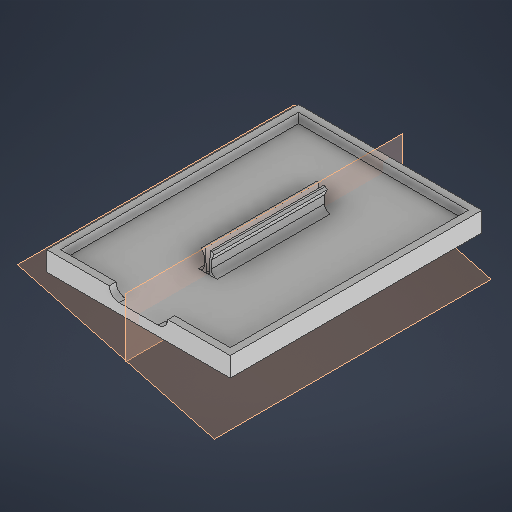
# Autodesk Inventor part: Bolt Slot Covers
Saved by Autodesk Inventor 2026.2 (Build 302298000, 298)
## iProperties
Created: 2026-05-27
Part Number: Bolt Slot Covers
Material: Generic
Document SubType Name: Modeling
Designer: mayhe
Density: 1 g/cm^3
Appearance: Default
Author: mayhe
Autodesk Inventor part; units mm, degrees
ref_plane "XZ Plane" through (0, 0, 0) normal (0, 1, 0) x (-1, 0, 0)
ref_plane "XY Plane" through (0, 0, 0) normal (0, 0, 1) x (1, 0, 0)
sketch "Sketch1" plane through (0, 0, 0) normal (0, 1, 0) x (-1, 0, 0)
  line L0 (47, 64.5) -> (-47, 64.5)
  line L1 (-47, 64.5) -> (-47, -64.5)
  line L2 (-47, -64.5) -> (47, -64.5)
  line L3 (47, -64.5) -> (47, 64.5)
  line L4 (47, 64.5) -> (-47, -64.5) construction
  line L5 (-47, 64.5) -> (47, -64.5) construction
  point P0 (0, 0)
  dimension "d0" = 94
  dimension "d1" = 129
  constraints: 12 end point, 2 midpoint, 2 parallel, 1 horizontal, 1 perpendicular
  measures "d0" distance of L2.end L1.end
  measures "d1" distance of L1.end L0.end
extrude "Base" add sketch "Sketch1" along normal mid plane 5
sketch "Sketch6" plane through (0, 2.5, 0) normal (0, 1, 0) x (1, 0, 0)
  line L0 (-47, -64.5) -> (47, -64.5) projected
  line L1 (-47, 64.5) -> (-47, -64.5) projected
  line L2 (-47, -64.5) -> (47, -64.5) projected
  line L3 (47, -64.5) -> (47, 64.5) projected
  line L4 (47, 64.5) -> (-47, 64.5) projected
  line L5 (-43.5, -61) -> (-43.5, 61)
  line L6 (-43.5, 61) -> (43.5, 61)
  line L7 (43.5, 61) -> (43.5, -61)
  line L8 (43.5, -61) -> (-43.5, -61)
  line L9 (0, -61) -> (0, -64.5)
  line L10 (-15, -61) -> (15, -61)
  line L11 (15, -61) -> (15, -64.5)
  line L12 (15, -64.5) -> (-15, -64.5)
  line L13 (-15, -64.5) -> (-15, -61)
  line L14 (-15, -61) -> (15, -64.5) construction
  line L15 (15, -61) -> (-15, -64.5) construction
  point P0 (0, 0)
  point P1 (0, -62.75)
  point P2 (-15, -61)
  point P3 (15, -61)
  point P4 (15, -64.5)
  point P5 (47, -64.5)
  dimension "d31" = 3.5
  dimension "d32" = 30
  constraints: 22 end point, 5 midpoint, 2 parallel, 1 horizontal, 1 perpendicular, 1 point on line, 3 other
  measures "d31" distance between parallel lines of L1 L5
  measures "d32" distance of L11.end L12.end
extrude "Walls" add sketch "Sketch6" along normal blind 5 contours L1 L4 L3 L0 L11 L8 L7 L6 L5 L13
sketch "Sketch7" plane through (0, 2.5, 0) normal (0, 1, 0) x (1, 0, 0)
  line L0 (0, 29) -> (0, -29) construction
  line L1 (-1.75, 29) -> (-1.75, -29)
  line L2 (1.75, -29) -> (1.75, 29)
  arc A0 (1.75, 29) -> (-1.75, 29) centre (0, 29) ccw
  arc A1 (-1.75, -29) -> (1.75, -29) centre (0, -29) ccw
  line L3 (1.75, -29) -> (-1.75, -29)
  line L4 (-1.75, 29) -> (1.75, 29)
  point P0 (0, 0)
  dimension "d35" = 29
  dimension "d36" = 3.5
  constraints: 12 end point, 4 point on circle, 4 tangent, 2 centre point, 2 parallel, 1 horizontal, 1 midpoint, 1 vertical
  measures "d35" distance of point (0, 0) L0.end
  measures "d36" diameter of A1
extrude "Extrusion7" add sketch "Sketch7" along normal blind 7 contours L4 L2 L3 L1
sketch "Sketch8" plane through (0, 9.5, 0) normal (0, 1, 0) x (1, 0, 0)
  line L0 (1.75, -29) -> (1.75, 29) projected
  line L1 (-1.75, 29) -> (-1.75, -29) projected
  arc A0 (-3.25, -29) -> (3.25, -29) centre (0, -29) ccw
  line L2 (-3.25, -29) -> (-3.25, 29)
  arc A1 (3.25, 29) -> (-3.25, 29) centre (0, 29) ccw
  line L3 (3.25, 29) -> (3.25, -29)
  line L4 (1.75, 29) -> (-1.75, 29) projected
  line L5 (-1.75, -29) -> (1.75, -29) projected
  line L6 (-3.25, -29) -> (3.25, -29)
  line L7 (-3.25, 29) -> (3.25, 29)
  point P0 (0, 0)
  constraints: 8 end point, 4 point on circle, 2 centre point, 1 horizontal, 1 parallel
extrude "Knob Width" add sketch "Sketch8" along normal blind 4 contours L5 L1 L4 L0 | L0 L7 L3 L6 | L6 L2 L7 L1
chamfer "Chamfer3" distance 1.5 distance2 3 2 edges at (-3.25, 9.5, 0) (3.25, 9.5, 0) measured on face at (2.75, 9.5, 0) measured on face at (-2.75, 9.5, 0)
chamfer "Chamfer4" distance 1 distance2 1 2 edges at (-3.25, 13.5, 0) (3.25, 13.5, 0) measured on face at (-2.75, 13.5, 0) measured on face at (2.75, 13.5, 0)
fillet "Fillet3" radius 3 2 edges at (1.75, 2.5, 0) (-1.75, 2.5, 0)
sketch "Sketch9" plane through (0, 13.5, 0) normal (0, 1, 0) x (1, 0, 0)
  line L0 (-0.625, 37.5) -> (0.625, 37.5)
  line L1 (0.625, 37.5) -> (0.625, -37.5)
  line L2 (0.625, -37.5) -> (-0.625, -37.5)
  line L3 (-0.625, 37.5) -> (0.625, -37.5) construction
  line L4 (0.625, 37.5) -> (-0.625, -37.5) construction
  line L5 (0, -32.25) -> (0, 0)
  line L6 (-1.75, 29) -> (-1.75, -29) projected
  line L7 (-0.625, -37.5) -> (-0.625, 37.5)
  point P0 (0.125, -28.4242)
  constraints: 14 end point, 3 parallel, 2 midpoint, 1 horizontal, 1 perpendicular
extrude "Extrusion9" cut sketch "Sketch9" against normal up to surface (11 mm away)
fillet "Fillet5" radius 5 2 edges at (-15, 2.5, 62.75) (15, 2.5, 62.75)
draft "FaceDraft4" angle 3.75 pull direction (0, 1, 0) faces at (-0.625, 9.8333, -9.6667) fixed edges at (-0.625, 2.5, 0)
draft "FaceDraft5" angle -3.75 pull direction (0, -1, 0) faces at (0.625, 9.8333, 9.6667) fixed edges at (0.625, 2.5, 0)
fillet "Fillet6" radius 0.5 2 edges at (-0.625, 2.5, 0) (0.625, 2.5, 0)
ref_plane "Work Plane1" through (-47, -2.5, -64.5) normal (0.258819, 0.9659258, 0) x (0, 0, -1)
sketch "Sketch10" plane through (-47, -2.5, -64.5) normal (0.258819, 0.9659258, 0) x (0, 0, -1)
  point P0 (-64.5, -44.7515)
body "Solid1"
